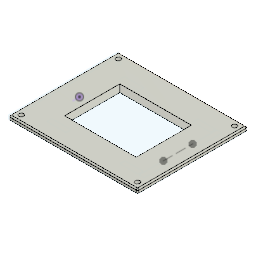
LCD Bezel 2.4in snap-in v1 (Autodesk Fusion 360 design; units mm, degrees)
Autodesk Fusion 360 part; units mm, degrees
sketch "Sketch1" plane through (0, 0, 0) normal (0, 0, 1) x (1, 0, 0)
  line L0 (-50.5, 43) -> (50.5, 43)
  line L1 (50.5, 43) -> (50.5, -43)
  line L2 (50.5, -43) -> (-50.5, -43)
  line L3 (-50.5, -43) -> (-50.5, 43)
  line L4 (-50.5, 43) -> (50.5, -43) construction
  line L5 (50.5, 43) -> (-50.5, -43) construction
  line L6 (25, 18.6) -> (-25, 18.6)
  line L7 (-25, 18.6) -> (-25, -18.6)
  line L8 (-25, -18.6) -> (25, -18.6)
  line L9 (25, -18.6) -> (25, 18.6)
  line L10 (25, 18.6) -> (-25, -18.6) construction
  line L11 (-25, 18.6) -> (25, -18.6) construction
  circle A0 centre (-45.5, 38) radius 5 construction
  circle A1 centre (-45.5, 38) radius 1.815
  line L12 (0, 55) -> (0, -45) construction
  line L13 (-60, 0) -> (80, 0) construction
  circle A2 centre (45.5, 38) radius 1.815
  circle A3 centre (45.5, -38) radius 1.815
  circle A4 centre (-45.5, -38) radius 1.815
  dimension "d1" = 101
  dimension "d2" = 86
  dimension "d3" = 50
  dimension "d4" = 37.2
  dimension "d5" = 5
  dimension "d6" = 3.63
  constraint perpendicular L0 L1
  constraint parallel L0 L2
  constraint parallel L1 L3
  constraint horizontal L0
  constraint coincident L4 origin
  constraint coincident L5 origin
  constraint perpendicular L6 L7
  constraint parallel L6 L8
  constraint parallel L7 L9
  constraint horizontal L6
  constraint coincident L10 origin
  constraint coincident L11 origin
  constraint tangent L3 A0
  constraint tangent L0 A0
  constraint concentric A0 A1
  constraint perpendicular L2 L12
  constraint perpendicular L3 L13
  constraint symmetric A1 L12 A2
  constraint symmetric A1 L13 A4
  constraint symmetric L13 A2 A3
  measures "d1" distance of L1.end L2.end
  measures "d2" distance of L0.end L1.end
  measures "d3" distance of L7.end L8.end
  measures "d4" distance of L6.end L7.end
  measures "d5" radius of A0
  measures "d6" diameter of A1
  measures "d14" distance of L0.start
extrude "Extrude1" add sketch "Sketch1" along normal blind 3
chamfer "Chamfer1" distance 3 angle 45 4 edges at (-25, 0, 3) (0, 18.6, 3) (25, 0, 3) (0, -18.6, 3)
sketch "Sketch2" plane through (-50.5, 0, 0) normal (-1, 0, 0) x (0, -1, 0)
  line L0 (-43, 0) -> (43, 0)
  line L1 (43, 0) -> (43, 3)
  line L2 (43, 3) -> (-43, 3)
  line L3 (-43, 3) -> (-43, 0)
fillet "Fillet1" radius 1 3 edges at (0, -43, 3) (0, 43, 3) (50.5, 0, 3)
sketch "Sketch3" plane through (0, 0, 0) normal (0, 0, 1) x (1, 0, 0)
  line L0 (-25.1574, -13.813) -> (-25.1574, 46.187) construction
  line L1 (25, 18.6) -> (25, -18.6)
  line L2 (25, -13.1739) -> (25, 45.4) construction
  line L3 (-34.0574, 33.1645) -> (-34.0574, -36.2651) construction
  line L4 (38.2, 40.4) -> (38.2, -34.6) construction
  line L5 (-25.1574, 18.7093) -> (64.6852, 18.7093) construction
  line L6 (60, 27.4093) -> (56.9479, 27.4093) construction
  line L7 (56.9479, 27.4093) -> (-67.0893, 27.4093) construction
  line L8 (60, -25.5) -> (-63.5008, -25.5) construction
  line L9 (25, -18.6) -> (-75, -18.6) construction
  line L10 (-34.0574, 0) -> (-37.9, 0)
  line L11 (-37.9, 0) -> (-37.9, -5)
  line L12 (-37.9, -5) -> (-34.0574, -5)
  line L13 (-34.0574, -5) -> (-34.0574, 0)
  line L14 (-34.0574, 0) -> (-38.0574, 0)
  line L15 (-38.0574, 0) -> (-38.0574, 5)
  line L16 (-38.0574, 5) -> (-34.0574, 5)
  line L17 (-34.0574, 5) -> (-34.0574, 0)
  line L18 (38.2, -25.5) -> (42.2, -25.5)
  line L19 (42.2, -25.5) -> (42.2, -10.5)
  line L20 (42.2, -10.5) -> (38.2, -10.5)
  line L21 (38.2, -10.5) -> (38.2, -25.5)
  line L22 (38.2, 27.4093) -> (42.2, 27.4093)
  line L23 (42.2, 27.4093) -> (42.2, 12.4093)
  line L24 (42.2, 12.4093) -> (38.2, 12.4093)
  line L25 (38.2, 12.4093) -> (38.2, 27.4093)
  line L26 (-34.0574, 27.4093) -> (-19.0574, 27.4093)
  line L27 (-19.0574, 27.4093) -> (-19.0574, 31.4093)
  line L28 (-19.0574, 31.4093) -> (-34.0574, 31.4093)
  line L29 (-34.0574, 31.4093) -> (-34.0574, 27.4093)
  line L30 (38.2, 27.4093) -> (23.2, 27.4093)
  line L31 (23.2, 27.4093) -> (23.2, 31.4093)
  line L32 (23.2, 31.4093) -> (38.2, 31.4093)
  line L33 (38.2, 31.4093) -> (38.2, 27.4093)
  line L34 (-34.0574, -25.5) -> (-19.0574, -25.5)
  line L35 (-19.0574, -25.5) -> (-19.0574, -29.5)
  line L36 (-19.0574, -29.5) -> (-34.0574, -29.5)
  line L37 (-34.0574, -29.5) -> (-34.0574, -25.5)
  line L38 (38.2, -25.5) -> (23.2, -25.5)
  line L39 (23.2, -25.5) -> (23.2, -29.5)
  line L40 (23.2, -29.5) -> (38.2, -29.5)
  line L41 (38.2, -29.5) -> (38.2, -25.5)
  line L42 (38.2, -25.5) -> (42.2, -25.5)
  line L43 (42.2, -25.5) -> (42.2, -29.5)
  line L44 (42.2, -29.5) -> (38.2, -29.5)
  line L45 (38.2, -29.5) -> (38.2, -25.5)
  line L46 (38.2, 27.4093) -> (42.2, 27.4093)
  line L47 (42.2, 27.4093) -> (42.2, 31.4093)
  line L48 (42.2, 31.4093) -> (38.2, 31.4093)
  line L49 (38.2, 31.4093) -> (38.2, 27.4093)
  dimension "d11" = 8.9
  dimension "d12" = 13.2
  dimension "d13" = 8.7
  dimension "d14" = 6.9
  dimension "d18" = 4
  dimension "d19" = 4
  dimension "d20" = 15
  dimension "d21" = 15
  dimension "d22" = 4
  dimension "d24" = 15
  dimension "d25" = 4
  dimension "d26" = 15
  dimension "d27" = 15
  dimension "d28" = 4
  dimension "d29" = 15
  dimension "d30" = 4
  dimension "d31" = 4
  dimension "d32" = 4
  dimension "d33" = 4
  dimension "d34" = 4
  dimension "d61" = 4
  constraint vertical L0
  constraint coincident L1 L2.start
  constraint parallel L1 L2
  constraint vertical L3
  constraint vertical L4
  constraint coincident L0 L5.start
  constraint perpendicular L0 L5
  constraint horizontal L6
  constraint parallel L6 L7
  constraint horizontal L8
  constraint coincident L1.end L9.start
  constraint perpendicular L1 L9
  constraint horizontal L10
  constraint vertical L11
  constraint horizontal L12
  constraint vertical L13
  constraint coincident L3 L10.start
  constraint horizontal L14
  constraint vertical L15
  constraint horizontal L16
  constraint vertical L17
  constraint horizontal L18
  constraint vertical L19
  constraint horizontal L20
  constraint vertical L21
  constraint coincident L4 L18.start
  constraint coincident L8 L18.start
  constraint horizontal L22
  constraint vertical L23
  constraint horizontal L24
  constraint vertical L25
  constraint coincident L4 L22.start
  constraint coincident L7 L22.start
  constraint horizontal L26
  constraint vertical L27
  constraint horizontal L28
  constraint vertical L29
  constraint coincident L3 L26.start
  constraint coincident L7 L26.start
  constraint horizontal L30
  constraint vertical L31
  constraint horizontal L32
  constraint vertical L33
  constraint horizontal L34
  constraint vertical L35
  constraint horizontal L36
  constraint vertical L37
  constraint coincident L3 L34.start
  constraint coincident L8 L34.start
  constraint horizontal L38
  constraint vertical L39
  constraint horizontal L40
  constraint vertical L41
  constraint horizontal L42
  constraint vertical L43
  constraint horizontal L44
  constraint vertical L45
  constraint horizontal L46
  constraint vertical L47
  constraint horizontal L48
  constraint vertical L49
  measures "d11" distance of L0 L3
  measures "d12" distance of L2 L4
  measures "d13" distance of L5 L7
  measures "d14" distance of L8 L9
  measures "d18" distance of L10.start L14.end
  measures "d19" distance of L18.start L18.end
  measures "d20" distance of L18.start L20.end
  measures "d21" distance of L22.start L24.end
  measures "d22" distance of L22.start L22.end
  measures "d24" distance of L26.start L26.end
  measures "d25" distance of L22.start L32.end
  measures "d26" distance of L22.start L30.end
  measures "d27" distance of L34.start L34.end
  measures "d28" distance of L34.start L36.end
  measures "d29" distance of L18.start L38.end
  measures "d30" distance of L18.start L40.end
  measures "d31" distance of L18.start L40.end
  measures "d32" distance of L18.start L18.end
  measures "d33" distance of L22.start L22.end
  measures "d34" distance of L22.start L32.end
  measures "d61" distance of L26 L28
extrude "Extrude2" add sketch "Sketch3" against normal blind 7.2
fillet "Fillet2" radius 1 2 edges at (50.5, 43, 1) (50.2071, 42.7071, 2.7071)
fillet "Fillet3" radius 1 2 edges at (50.5, -43, 1) (50.2071, -42.7071, 2.7071)
fillet "Fillet4" radius 1 5 edges at (-50.5, 43, 1) (-50.5, 42.7071, 2.7071) (-50.5, 0, 3) (-50.5, -42.7071, 2.7071) (-50.5, -43, 1)
sketch "Sketch4" plane through (0, -25.5, 0) normal (0, 1, 0) x (-1, 0, 0)
  line L0 (-23.2, 0) -> (-38.2, 0)
  line L1 (-38.2, 0) -> (-38.2, -7.2)
  line L2 (-38.2, -7.2) -> (-23.2, -7.2)
  line L3 (-23.2, -7.2) -> (-23.2, 0)
  line L4 (-23.2, -7.2) -> (-38.2, -7.2)
  line L5 (-38.2, -7.2) -> (-38.2, -6.2)
  line L6 (-38.2, -6.2) -> (-23.2, -6.2)
  line L7 (-23.2, -6.2) -> (-23.2, -7.2)
  dimension "d40" = 1
  constraint horizontal L4
  constraint vertical L5
  constraint horizontal L6
  constraint vertical L7
  constraint coincident L2.end L3.start
  measures "d40" distance of L2.end L6.end
sketch "Sketch5" plane through (0, -25.5, 0) normal (0, 1, 0) x (-1, 0, 0)
  line L0 (34.0574, 0) -> (19.0574, 0)
  line L1 (19.0574, 0) -> (19.0574, -7.2)
  line L2 (19.0574, -7.2) -> (34.0574, -7.2)
  line L3 (34.0574, -7.2) -> (34.0574, 0)
  line L4 (34.0574, -7.2) -> (19.0574, -7.2)
  line L5 (19.0574, -7.2) -> (19.0574, -6.2)
  line L6 (19.0574, -6.2) -> (34.0574, -6.2)
  line L7 (34.0574, -6.2) -> (34.0574, -7.2)
  dimension "d43" = 1
  constraint horizontal L4
  constraint vertical L5
  constraint horizontal L6
  constraint vertical L7
  constraint coincident L2.end L3.start
  measures "d43" distance of L2.end L6.end
extrude "Extrude4" add sketch "Sketch5" along normal blind 1 contours L1 L2 L3 L4 L5 L6 L7
sketch "Sketch6" plane through (0, 27.4093, 0) normal (0, -1, 0) x (1, 0, 0)
  line L0 (-19.0574, 0) -> (-34.0574, 0)
  line L1 (-34.0574, 0) -> (-34.0574, -7.2)
  line L2 (-34.0574, -7.2) -> (-19.0574, -7.2)
  line L3 (-19.0574, -7.2) -> (-19.0574, 0)
  line L4 (-19.0574, -7.2) -> (-34.0574, -7.2)
  line L5 (-34.0574, -7.2) -> (-34.0574, -6.2)
  line L6 (-34.0574, -6.2) -> (-19.0574, -6.2)
  line L7 (-19.0574, -6.2) -> (-19.0574, -7.2)
  dimension "d46" = 1
  constraint horizontal L4
  constraint vertical L5
  constraint horizontal L6
  constraint vertical L7
  constraint coincident L1 L5.end
  constraint coincident L2.end L3.start
  measures "d46" distance of L2.end L6.end
extrude "Extrude5" add sketch "Sketch6" along normal blind 1 contours L1 L2 L3 L4 L5 L6 L7
sketch "Sketch7" plane through (0, 0, -7.2) normal (0, 0, -1) x (1, 0, 0)
  line L0 (42.2, -31.4093) -> (42.2, -12.4093)
  line L1 (42.2, -12.4093) -> (38.2, -12.4093)
  line L2 (38.2, -12.4093) -> (38.2, -27.4093)
  line L3 (38.2, -27.4093) -> (23.2, -27.4093)
  line L4 (23.2, -27.4093) -> (23.2, -31.4093)
  line L5 (23.2, -31.4093) -> (42.2, -31.4093)
  line L6 (38.2, -27.4093) -> (37.2, -27.4093)
  line L7 (37.2, -27.4093) -> (37.2, -31.4093)
  line L8 (37.2, -31.4093) -> (38.2, -31.4093)
  line L9 (38.2, -31.4093) -> (38.2, -27.4093)
  dimension "d49" = 1
  constraint horizontal L6
  constraint vertical L7
  constraint horizontal L8
  constraint vertical L9
  constraint coincident L2.end L3.start
  measures "d49" distance of L2.end L6.end
extrude "Extrude6" cut sketch "Sketch7" against normal up to surface (7.2 mm away) contours L3 L5 L6 L7 L8 L9
sketch "Sketch8" plane through (0, 0, -7.2) normal (0, 0, -1) x (1, 0, 0)
  line L0 (42.2, 10.5) -> (42.2, 29.5)
  line L1 (42.2, 29.5) -> (23.2, 29.5)
  line L2 (23.2, 29.5) -> (23.2, 25.5)
  line L3 (23.2, 25.5) -> (38.2, 25.5)
  line L4 (38.2, 25.5) -> (38.2, 10.5)
  line L5 (38.2, 10.5) -> (42.2, 10.5)
  line L6 (38.2, 25.5) -> (37.2, 25.5)
  line L7 (37.2, 25.5) -> (37.2, 29.5)
  line L8 (37.2, 29.5) -> (38.2, 29.5)
  line L9 (38.2, 29.5) -> (38.2, 25.5)
  dimension "d52" = 1
  constraint horizontal L6
  constraint vertical L7
  constraint horizontal L8
  constraint vertical L9
  constraint coincident L3.end L4.start
  measures "d52" distance of L3.end L6.end
extrude "Extrude7" cut sketch "Sketch8" against normal up to surface (7.2 mm away) contours L1 L3 L6 L7 L8 L9
sketch "Sketch9" plane through (0, -25.5, 0) normal (0, 1, 0) x (-1, 0, 0)
  line L0 (-37.2, 0) -> (-37.2, -7.2)
  line L1 (-37.2, -7.2) -> (-23.2, -7.2)
  line L2 (-23.2, -7.2) -> (-23.2, 0)
  line L3 (-23.2, 0) -> (-37.2, 0)
  line L4 (-23.2, -7.2) -> (-37.2, -7.2)
  line L5 (-37.2, -7.2) -> (-37.2, -6.2)
  line L6 (-37.2, -6.2) -> (-23.2, -6.2)
  line L7 (-23.2, -6.2) -> (-23.2, -7.2)
  dimension "d55" = 1
  constraint horizontal L4
  constraint vertical L5
  constraint horizontal L6
  constraint vertical L7
  constraint coincident L1.end L2.start
  measures "d55" distance of L1.end L6.end
extrude "Extrude8" add sketch "Sketch9" along normal blind 1 contours L0 L1 L2 L4 L5 L6 L7
sketch "Sketch10" plane through (0, 27.4093, 0) normal (0, -1, 0) x (1, 0, 0)
  line L0 (37.2, -7.2) -> (37.2, 0)
  line L1 (37.2, 0) -> (23.2, 0)
  line L2 (23.2, 0) -> (23.2, -7.2)
  line L3 (23.2, -7.2) -> (37.2, -7.2)
  line L4 (23.2, -7.2) -> (37.2, -7.2)
  line L5 (37.2, -7.2) -> (37.2, -6.2)
  line L6 (37.2, -6.2) -> (23.2, -6.2)
  line L7 (23.2, -6.2) -> (23.2, -7.2)
  dimension "d58" = 1
  constraint horizontal L4
  constraint vertical L5
  constraint horizontal L6
  constraint vertical L7
  constraint coincident L2.end L3.start
  measures "d58" distance of L2.end L6.end
extrude "Extrude9" add sketch "Sketch10" along normal blind 1 contours L0 L2 L3 L4 L5 L6 L7
sketch "Sketch11" plane through (0, 0, 0) normal (0, 0, -1) x (1, 0, 0)
  line L0 (38.2, 29.5) -> (42.2, 29.5)
  line L1 (42.2, 29.5) -> (42.2, 10.5)
  line L2 (42.2, 10.5) -> (38.2, 10.5)
  line L3 (38.2, 10.5) -> (38.2, 29.5)
  line L4 (38.2, -31.4093) -> (38.2, -12.4093)
  line L5 (38.2, -12.4093) -> (42.2, -12.4093)
  line L6 (42.2, -12.4093) -> (42.2, -31.4093)
  line L7 (42.2, -31.4093) -> (38.2, -31.4093)
  arc A0 (-50.5, -42) -> (-49.5, -43) centre (-49.5, -42) ccw
  line L8 (-49.5, -43) -> (49.5, -43)
  arc A1 (49.5, -43) -> (50.5, -42) centre (49.5, -42) ccw
  line L9 (50.5, -42) -> (50.5, 42)
  arc A2 (50.5, 42) -> (49.5, 43) centre (49.5, 42) ccw
  line L10 (49.5, 43) -> (-49.5, 43)
  arc A3 (-49.5, 43) -> (-50.5, 42) centre (-49.5, 42) ccw
  line L11 (-50.5, 42) -> (-50.5, -42)
  line L12 (-37.9, 5) -> (-34.0574, 5)
  line L13 (-34.0574, 5) -> (-34.0574, -5)
  line L14 (-34.0574, -5) -> (-38.0574, -5)
  line L15 (-38.0574, -5) -> (-38.0574, 0)
  line L16 (-19.0574, 29.5) -> (-19.0574, 25.5)
  line L17 (-19.0574, 25.5) -> (-34.0574, 25.5)
  line L18 (-34.0574, 25.5) -> (-34.0574, 29.5)
  line L19 (-34.0574, 29.5) -> (-19.0574, 29.5)
  line L20 (-34.0574, -27.4093) -> (-19.0574, -27.4093)
  line L21 (-19.0574, -27.4093) -> (-19.0574, -31.4093)
  line L22 (-19.0574, -31.4093) -> (-34.0574, -31.4093)
  line L23 (-34.0574, -31.4093) -> (-34.0574, -27.4093)
  line L24 (37.2, 29.5) -> (37.2, 25.5)
  line L25 (37.2, 25.5) -> (23.2, 25.5)
  line L26 (23.2, 25.5) -> (23.2, 29.5)
  line L27 (23.2, 29.5) -> (37.2, 29.5)
  line L28 (37.2, -27.4093) -> (37.2, -31.4093)
  line L29 (37.2, -31.4093) -> (23.2, -31.4093)
  line L30 (23.2, -31.4093) -> (23.2, -27.4093)
  line L31 (23.2, -27.4093) -> (37.2, -27.4093)
  circle A4 centre (-45.5, 38) radius 1.815
  line L32 (25, 18.6) -> (25, -18.6)
  line L33 (25, -18.6) -> (-25, -18.6)
  line L34 (-25, -18.6) -> (-25, 18.6)
  line L35 (-25, 18.6) -> (25, 18.6)
  circle A5 centre (45.5, 38) radius 1.815
  circle A6 centre (-45.5, -38) radius 1.815
  circle A7 centre (45.5, -38) radius 1.815
  line L36 (38.2, 10.5) -> (38.2, -12.4093) construction
  line L37 (-38.0574, 0) -> (-37.9, 0)
  line L38 (-37.9, 0) -> (-37.9, 5)
  constraint coincident L2.end L3.start
  constraint coincident L4.end L5.start
fillet "Fillet5" radius 0.3 1 edges at (-26.5574, -24.5, -7.2)
fillet "Fillet6" radius 0.3 3 edges at (-26.5574, 26.4093, -7.2) (30.2, 26.4093, -7.2) (30.2, -24.5, -7.2)
